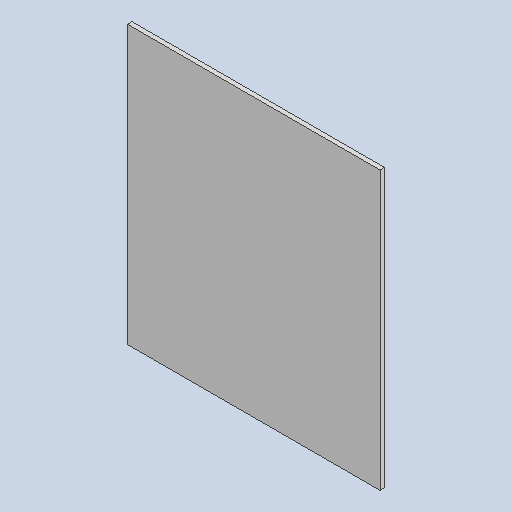
# Autodesk Inventor part: Part7
Saved by Autodesk Inventor 2023 (Build 270158000, 158)
## iProperties
Created: 2024-03-19
Part Number: Part7
Material: Generic
Document SubType Name: Modeling
Designer: noname
Density: 1 g/cm^3
Appearance: Default
Author: noname
Autodesk Inventor part; units mm, degrees
ref_plane "YZ Plane" through (0, 0, 0) normal (1, 0, 0) x (0, 1, 0)
ref_plane "XZ Plane" through (0, 0, 0) normal (0, 1, 0) x (-1, 0, 0)
ref_plane "XY Plane" through (0, 0, 0) normal (0, 0, 1) x (1, 0, 0)
sketch "Sketch1" plane through (0, 0, 0) normal (0, 0, 1) x (1, 0, 0)
  line L0 (-49.5, 42.5) -> (-49.5, -45.5) projected
  line L1 (-49.5, -45.5) -> (41.5, -45.5) projected
  line L2 (41.5, -45.5) -> (41.5, 42.5) projected
  line L3 (41.5, 42.5) -> (-49.5, 42.5) projected
  line L4 (-49.5, 42.5) -> (41.5, 42.5)
  line L5 (41.5, 42.5) -> (41.5, -57.5)
  line L6 (41.5, -57.5) -> (-49.5, -57.5)
  line L7 (-49.5, -57.5) -> (-49.5, 42.5)
  line L8 (42.73, 27.5) -> (60.73, 27.5)
  line L9 (60.73, 27.5) -> (60.73, 9.5)
  line L10 (60.73, 9.5) -> (42.73, 9.5)
  line L11 (42.73, 9.5) -> (42.73, 27.5)
  line L12 (42.73, -10.5) -> (42.73, 7.5)
  line L13 (60.73, -10.5) -> (42.73, -10.5)
  line L14 (60.73, 7.5) -> (60.73, -10.5)
  line L15 (42.73, 7.5) -> (60.73, 7.5)
  line L16 (42.73, -30.5) -> (42.73, -12.5)
  line L17 (60.73, -30.5) -> (42.73, -30.5)
  line L18 (60.73, -12.5) -> (60.73, -30.5)
  line L19 (42.73, -12.5) -> (60.73, -12.5)
  line L20 (41.5, 42.5) -> (50.5, 29.4671)
  line L21 (50.5, 29.4671) -> (50.5, -32.4671)
  line L22 (50.5, -32.4671) -> (41.5, -45.5)
  line L23 (0.5, -35) -> (-8.5, -35) projected
  line L24 (-8.5, -35) -> (-8.5, 32) projected
  line L25 (-8.5, 32) -> (0.5, 32) projected
  line L26 (0.5, 32) -> (0.5, -35) projected
  line L27 (-17.5, -35) -> (-26.5, -35) projected
  line L28 (-26.5, -35) -> (-26.5, 32) projected
  line L29 (-26.5, 32) -> (-17.5, 32) projected
  line L30 (-17.5, 32) -> (-17.5, -35) projected
  line L31 (18.5, -35) -> (9.5, -35) projected
  line L32 (9.5, -35) -> (9.5, 32) projected
  line L33 (9.5, 32) -> (18.5, 32) projected
  line L34 (18.5, 32) -> (18.5, -35) projected
  line L35 (-35.5, -35) -> (-44.5, -35) projected
  line L36 (-44.5, -35) -> (-44.5, 32) projected
  line L37 (-44.5, 32) -> (-35.5, 32) projected
  line L38 (-35.5, 32) -> (-35.5, -35) projected
  line L39 (36.5, -35) -> (27.5, -35) projected
  line L40 (27.5, -35) -> (27.5, 32) projected
  line L41 (27.5, 32) -> (36.5, 32) projected
  line L42 (36.5, 32) -> (36.5, -35) projected
  point P0 (0, 0)
  point P1 (-38.5, -35)
  point P2 (-41.5, -35)
  point P3 (-41.5, 32)
  point P4 (-38.5, 32)
  point P5 (-20.5, -35)
  point P6 (-23.5, -35)
  point P7 (-23.5, 32)
  point P8 (-20.5, 32)
  point P9 (-2.5, -35)
  point P10 (-5.5, -35)
  point P11 (-5.5, 32)
  point P12 (-2.5, 32)
  point P13 (15.5, -35)
  point P14 (12.5, -35)
  point P15 (12.5, 32)
  point P16 (15.5, 32)
  point P17 (33.5, -35)
  point P18 (30.5, -35)
  point P19 (30.5, 32)
  point P20 (33.5, 32)
  point P21 (41.5, -45.5)
  point P22 (-49.5, -45.5)
  point P23 (60.73, -1.5)
  point P24 (50.5, -1.5)
  dimension "d0" = 100
  dimension "d6" = 20
  dimension "d12" = 100
  dimension "d13" = 18
  constraints: 38 end point, 4 parallel, 2 equal length, 2 horizontal, 2 midpoint, 2 perpendicular, 2 vertical, 1 horizontal alignment, 16 other
  measures "d0" distance between parallel lines of L6 L3
  measures "d6" distance of L8.start L12.end
  measures "d12" distance between parallel lines of L0 L21
  measures "d13" distance between parallel lines of L10 L8
extrude "Extrusion1" add sketch "Sketch1" along normal blind 1.6 contours L3 L2 L1 L0 | L1 L5 L6 L7 | L23 L24 L25 L26 | L27 L28 L29 L30 | L31 L32 L33 L34 | L35 L36 L37 L38 | L39 L40 L41 L42
body "Solid1"
